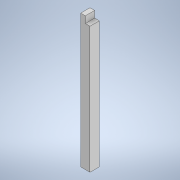
# Autodesk Inventor part: Columna
Saved by Autodesk Inventor 2022 (Build 260153000, 153)
## iProperties
Created: 2022-01-21
Part Number: Columna
Material: Generic
Document SubType Name: Modeling
Designer: galug
Density: 1 g/cm^3
Appearance: Default
Author: galug
Autodesk Inventor part; units mm, degrees
ref_plane "YZ Plane" through (0, 0, 0) normal (1, 0, 0) x (0, 1, 0)
ref_plane "XZ Plane" through (0, 0, 0) normal (0, 1, 0) x (-1, 0, 0)
ref_plane "XY Plane" through (0, 0, 0) normal (0, 0, 1) x (1, 0, 0)
sketch "Base" plane through (0, 0, 0) normal (0, 1, 0) x (-1, 0, 0)
  line L0 (350, 350) -> (-350, 350)
  line L1 (-350, 350) -> (-350, -350)
  line L2 (-350, -350) -> (350, -350)
  line L3 (350, -350) -> (350, 350)
  line L4 (350, 350) -> (-350, -350) construction
  line L5 (-350, 350) -> (350, -350) construction
  point P0 (0, 0)
  dimension "d0" = 700
  dimension "d1" = 700
  constraints: 12 end point, 2 midpoint, 2 parallel, 1 horizontal, 1 perpendicular
  measures "d0" distance of L2.end L1.end
  measures "d1" distance of L1.end L0.end
extrude "Extrusion1" add sketch "Base" along normal blind 10000
sketch "CortePoleas" plane through (0, 10000, 0) normal (0, 1, 0) x (1, 0, 0)
  line L0 (350, 350) -> (-350, 350) projected
  line L1 (350, -350) -> (350, 350) projected
  line L2 (0, 350) -> (350, 350)
  line L3 (350, 350) -> (350, -350)
  line L4 (350, -350) -> (0, -350)
  line L5 (0, -350) -> (0, 350)
  point P0 (0, 0)
  constraints: 8 end point, 2 parallel, 1 horizontal, 1 midpoint, 1 perpendicular
extrude "Extrusion2" cut sketch "CortePoleas" against normal blind 500
body "Solid1"
